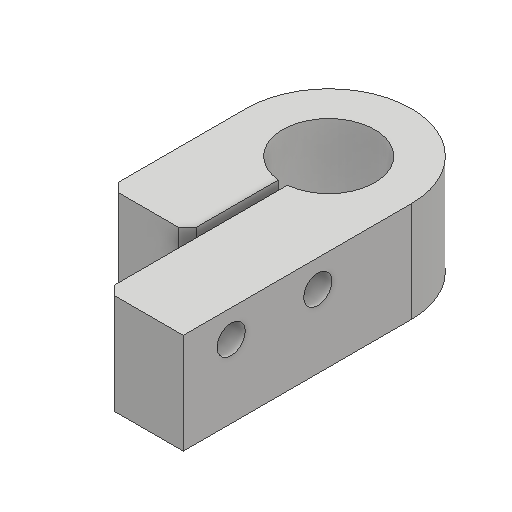
# Autodesk Inventor part: 3DP_ABS_X_Axis_Endstop_Mount
Saved by Autodesk Inventor 2026.1 (Build 301233000, 233)
## iProperties
Created: 2017-05-28
Part Number: 3DP_ABS_X_Axis_Endstop_Mount
Material: Ogólny
Document SubType Name: Modeling
Designer: Andrzej
Density: 1 g/cm^3
Appearance: Domyślna
Mass: 4.14123 g
Surface Area: 25.8164 cm^2
Volume: 4.14123 cm^3
Author: Andrzej
Autodesk Inventor part; units mm, degrees
ref_plane "YZ Plane" through (0, 0, 0) normal (1, 0, 0) x (0, 1, 0)
ref_plane "XZ Plane" through (0, 0, 0) normal (0, 1, 0) x (-1, 0, 0)
ref_plane "XY Plane" through (0, 0, 0) normal (0, 0, 1) x (1, 0, 0)
sketch "Szkic1" plane through (0, 0, 0) normal (0, 0, 1) x (1, 0, 0)
  arc A0 (0.5, -5.0252) -> (-0.5, -5.0252) centre (0, 0) ccw
  arc A1 (0.5, -9.0362) -> (-0.5, -9.0362) centre (0, 0) ccw
  line L0 (-9.05, 0) -> (-9.05, -25)
  line L1 (-9.05, -25) -> (-0.5, -25)
  line L2 (9.05, 0) -> (9.05, -25)
  line L3 (9.05, -25) -> (0.5, -25)
  line L4 (-0.5, -25) -> (-0.5, -5.0252)
  line L5 (0.5, -25) -> (0.5, -5.0252)
  dimension "d0" = 10.1
  dimension "d1" = 4
  dimension "d2" = 8.55
  dimension "d3" = 8.55
  dimension "d4" = 25
  dimension "d5" = 25
  dimension "d7" = 1
  constraints: 12 end point, 6 point on circle, 4 point on line, 2 centre point, 2 vertical, 1 coincident, 1 parallel, 1 perpendicular, 1 tangent
  measures "d0" diameter of A0
  measures "d1" radial gap between concentric circles of A0 A1
  measures "d2" distance of L0.end L1.end
  measures "d3" distance of L2.end L3.end
  measures "d4" distance of L2.start L2.end
  measures "d5" distance of L0.start L0.end
  measures "d7" distance between parallel lines of L5 L4
extrude "Wyciągnięcie proste1" add sketch "Szkic1" along normal blind 11
sketch "Szkic2" plane through (9.05, -25, 0) normal (1, 0, 0) x (0, 0, -1)
  line L0 (0, 0) -> (0, 25) projected
  line L1 (0, 25) -> (-11, 25) projected
  line L2 (-11, 0) -> (-11, 25) projected
  line L3 (0, 0) -> (-11, 0) projected
  line L4 (0, 20) -> (-11, 20)
  line L5 (-11, 25) -> (-11, 0) projected
  point P0 (-8, 5.25)
  point P1 (-8, 14.75)
  dimension "d10" = 5.25
  dimension "d11" = 20
  dimension "d12" = 5.25
  dimension "d13" = 11
  dimension "d14" = 3
  dimension "d15" = 3
  constraints: 2 end point, 2 point on line, 1 perpendicular
  measures "d10" distance from line of L3 point (-8, 5.25)
  measures "d11" distance between parallel lines of L3 L4
  measures "d12" distance from line of L4 point (-8, 14.75)
  measures "d13" distance between parallel lines of L0 L2
  measures "d14" distance from line of L2 point (-8, 14.75)
  measures "d15" distance from line of L2 point (-8, 5.25)
hole "Otwór1" at (9.05, -19.75, 8) at (9.05, -10.25, 8) direction (-1, 0, 0) diameter 3.1 end through all
sketch "Szkic3" plane through (-9.05, -25, 0) normal (0, -1, 0) x (1, 0, 0)
  line L0 (0, 0) -> (8.55, 0) projected
  line L1 (8.55, 0) -> (8.55, 11) projected
  line L2 (0, 11) -> (8.55, 11) projected
  line L3 (0, 0) -> (0, 11) projected
  point P0 (9.05, 0)
extrude "Wyciągnięcie proste2" cut sketch "Szkic3" against normal blind 10
chamfer "Faza1" distance 1 angle 45 3 edges at (-9.05, -15, 5.5) (-0.5, -15, 5.5) (0.5, -25, 5.5)
equation "\"d3\" = d2"
equation "\"d4\" = d5"
